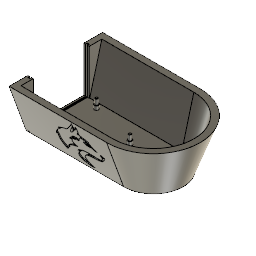
BlimpEnclosure v6 (Autodesk Fusion 360 design; units mm, degrees)
Autodesk Fusion 360 part; units mm, degrees
sketch "Sketch1" plane through (0, 0, 0) normal (0, 0, 1) x (1, 0, 0)
  line L0 (0, -53.3) -> (0, 0)
  circle A0 centre (15.3, -2.6) radius 1.4
  circle A1 centre (14, -50.8) radius 1.4
  circle A2 centre (66.1, -17.8) radius 1.4
  circle A3 centre (66.1, -45.7) radius 1.4
  line L1 (100, -58.3) -> (0, -58.3)
  line L2 (0, -58.3) -> (0, 5)
  line L3 (0, 5) -> (100, 5)
  line L4 (100, 5) -> (100, -58.3)
  line L5 (100, -58.3) -> (0, 5) construction
  line L6 (0, -58.3) -> (100, 5) construction
  arc A4 (100, -58.3) -> (100, 5) centre (100, -26.65) ccw
  line L7 (2, 3) -> (100, 3)
  arc A5 (100, -56.3) -> (100, 3) centre (100, -26.65) ccw
  line L8 (100, -56.3) -> (2, -56.3)
  line L9 (2, -56.3) -> (2, 3)
  line L10 (2, 3) -> (2, 5)
  line L11 (2, -56.3) -> (2, -58.3)
  point P0 (50, -26.65)
  dimension "d3" = 2.8
  dimension "d7" = 2.8
  dimension "d8" = 2.8
  dimension "d9" = 2.8
  dimension "d19" = 100
  dimension "d20" = 63.3
  dimension "d21" = 2
  constraint vertical L0
  constraint coincident L0.end origin
  constraint perpendicular L1 L2
  constraint parallel L1 L3
  constraint parallel L2 L4
  constraint horizontal L1
  constraint coincident L5 P0
  constraint coincident L6 P0
  constraint tangent L1 A4
  constraint coincident L3 L10.end
  constraint perpendicular L3 L10
  constraint coincident L1 L11.end
  constraint perpendicular L1 L11
  measures "d3" diameter of A0
  measures "d7" diameter of A1
  measures "d8" diameter of A2
  measures "d9" diameter of A3
  measures "d19" distance of L2.end L3.end
  measures "d20" distance of L1.end L2.end
extrude "Extrude1" add sketch "Sketch1" along normal blind 2 contours L4 L7 L8 L9 | L4 A5 makes body 1
extrude "Extrude2" add sketch "Sketch1" along normal blind 12 contours A0 | A1 | A2 | A3 bodies 1
sketch "Sketch2" plane through (0, 0, 2) normal (0, 0, 1) x (-1, 0, 0)
  circle A0 centre (-15.3, 2.6) radius 1.4
  circle A1 centre (-66.1, 17.8) radius 1.4
  circle A2 centre (-14, 50.8) radius 1.4
  circle A3 centre (-66.1, 45.7) radius 1.4
  arc A4 (-100, 56.3) -> (-100, -3) centre (-100, 26.65) ccw
  line L0 (-100, -3) -> (-2, -3)
  line L1 (-2, -3) -> (-2, 56.3)
  line L2 (-2, 56.3) -> (-100, 56.3)
  circle A5 centre (-15.3, 2.6) radius 2.25
  circle A6 centre (-66.1, 17.8) radius 2.25
  circle A7 centre (-66.1, 45.7) radius 2.25
  circle A8 centre (-14, 50.8) radius 2.25
  dimension "d26" = 4.5
  dimension "d27" = 4.5
  dimension "d28" = 4.5
  dimension "d29" = 4.5
  constraint concentric A0 A5
  constraint concentric A1 A6
  constraint concentric A3 A7
  constraint concentric A2 A8
  measures "d26" diameter of A5
  measures "d27" diameter of A6
  measures "d28" diameter of A7
  measures "d29" diameter of A8
extrude "Extrude3" add sketch "Sketch2" along normal blind 4 separate body contours A5 | A6 | A7 | A8 makes body 2 at (68.2143, -46.4695, 4.6667) makes body 3 at (11.7612, -50.576, 4.6667) makes body 4 at (63.8612, -17.576, 4.6667) makes body 5 at (13.0612, -2.376, 4.6667)
chamfer "Chamfer1" distance 0.4 angle 45 4 edges at (13.9947, -3.1063, 12) (64.7947, -18.3063, 12) (64.7947, -46.2063, 12) (12.6947, -51.3063, 12) on bodies 1
extrude "Extrude4" add sketch "Sketch1" along normal blind 50 separate body contours L1 L4 L8 L11 | L3 L4 L7 L10 | L4 A4 A5 makes body 6
draft "Draft1" angle 20 neutral plane through (0, 0, 0) pull (0, 0, -1) 3 faces at (115.1367, 1.1457, 16.6667) (34.6667, 5, 16.6667) (67.3333, -58.3, 16.6667) on bodies 6
extrude "Extrude5" add sketch "Sketch1" along normal blind 1 contours L0 L1 L2 L3 L9 L10 L11 bodies 1 6
extrude "Extrude6" add 1 faces at (2, -63.0328, 34) along direction (-1, 0, 0) blind 4 separate body on bodies 1 makes body 7
extrude "Extrude7" add 1 faces at (0, -37.2, 0.3333) along direction (-1, 0, 0) blind 2 separate body on bodies 1 makes body 8
extrude "Extrude8" cut 1 faces at (1.3333, -37.2, 1) along direction (0, 0, 1) blind 49 on bodies 1 bodies 7
draft "Draft2" angle -15 neutral plane through (0, 0, 0) pull (0, 0, -1) 3 faces at (102.9522, 2.8527, 34) (67.3333, -56.3, 18) (34.6667, 3, 18) on bodies 1
extrude "Extrude9" add 1 faces at (1.3333, -37.2, 1) along direction (0, 0, 1) blind 49 on bodies 1 bodies 1 7 8
extrude "Extrude10" add 1 faces at (-2, -63.0328, 34) along direction (-1, 0, 0) blind 2 on bodies 1 bodies 1
sketch "Sketch3" plane through (0, 0, 50) normal (0, 0, 1) x (-1, 0, 0)
  line L0 (4, 76.4985) -> (-100, 76.4985)
  arc A0 (-100, 76.4985) -> (-100, -23.1985) centre (-100, 26.65) ccw
  line L1 (-100, -23.1985) -> (4, -23.1985)
  line L2 (4, -23.1985) -> (4, -3)
  line L3 (4, -3) -> (0, -3)
  line L4 (0, -3) -> (0, 56.3)
  line L5 (0, 56.3) -> (4, 56.3)
  line L6 (4, 56.3) -> (4, 76.4985)
  line L7 (-2, 69.6975) -> (-2, -16.3975)
  line L8 (-2, -16.3975) -> (-100, -16.3975)
  arc A1 (-100, 69.6975) -> (-100, -16.3975) centre (-100, 26.65) ccw
  line L9 (-100, 69.6975) -> (-2, 69.6975)
  line L10 (0, -3) -> (-2, -3)
  line L11 (0, 56.3) -> (-2, 56.3)
  line L12 (2, -5) -> (0, -5)
  line L13 (0, -5) -> (0, 58)
  line L14 (0, 58) -> (2, 58)
  line L15 (2, 58) -> (2, -5)
  point P0 (-2, -3)
  point P1 (-2, 56.3)
  constraint coincident L3.end L4.start
  constraint coincident P0 L10.end
  constraint coincident L4.end L5.start
  constraint coincident P1 L11.end
  constraint horizontal L12
  constraint vertical L13
  constraint horizontal L14
  constraint vertical L15
sketch "Sketch4" plane through (0, 0, 50) normal (0, 0, 1) x (-1, 0, 0)
  line L0 (4, 76.4985) -> (-100, 76.4985)
  arc A0 (-100, 76.4985) -> (-100, -23.1985) centre (-100, 26.65) ccw
  line L1 (-100, -23.1985) -> (4, -23.1985)
  line L2 (4, -23.1985) -> (4, -3)
  line L3 (4, -3) -> (0, -3)
  line L4 (0, -3) -> (0, 56.3)
  line L5 (0, 56.3) -> (4, 56.3)
  line L6 (4, 56.3) -> (4, 76.4985)
  line L7 (-2, 69.6975) -> (-2, -16.3975)
  line L8 (-2, -16.3975) -> (-100, -16.3975)
  arc A1 (-100, 69.6975) -> (-100, -16.3975) centre (-100, 26.65) ccw
  line L9 (-100, 69.6975) -> (-2, 69.6975)
sketch "Sketch5" plane through (2, 0, 0) normal (1, 0, 0) x (0, 1, 0)
  line L0 (3.5359, 2) -> (16.3975, 50)
  line L1 (16.3975, 50) -> (-69.6975, 50)
  line L2 (-69.6975, 50) -> (-56.8359, 2)
  line L3 (-56.8359, 2) -> (3.5359, 2)
  line L4 (3, 50) -> (3, 2)
  line L5 (-56.3, 50) -> (-56, 2)
  line L6 (3, 50) -> (-56.3, 50)
  line L7 (3, 2) -> (-56, 2)
  line L8 (3, 50) -> (-56.3, 50)
  line L9 (-56.3, 50, -2) -> (3, 50, -2)
  line L10 (3, 50, -2) -> (3, 2, 0)
  point P0 (3, 50)
  point P1 (-56.3, 50)
  point P2 (-56.3, 50)
  point P3 (3, 50)
  constraint coincident P3 P0
  constraint coincident L3 L4.end
  constraint coincident P2 P1
  constraint coincident L3 L5.end
sketch "Sketch6" plane through (0, 0, 50) normal (0, 0, 1) x (-1, 0, 0)
  line L0 (4, 76.4985) -> (-100, 76.4985)
  arc A0 (-100, 76.4985) -> (-100, -23.1985) centre (-100, 26.65) ccw
  line L1 (-100, -23.1985) -> (4, -23.1985)
  line L2 (4, -23.1985) -> (4, -3)
  line L3 (4, -3) -> (0, -3)
  line L4 (0, -3) -> (0, 56.3)
  line L5 (0, 56.3) -> (4, 56.3)
  line L6 (4, 56.3) -> (4, 76.4985)
  line L7 (-2, 69.6975) -> (-2, -16.3975)
  line L8 (-2, -16.3975) -> (-100, -16.3975)
  arc A1 (-100, 69.6975) -> (-100, -16.3975) centre (-100, 26.65) ccw
  line L9 (-100, 69.6975) -> (-2, 69.6975)
  line L10 (-2, 56.3) -> (0, 56.3)
  line L11 (0, 56.3) -> (0, -3)
  line L12 (0, -3) -> (-2, -3)
  line L13 (-2, -3) -> (-2, 56.3)
  point P0 (-2, 56.3)
  constraint horizontal L10
  constraint vertical L11
  constraint horizontal L12
  constraint vertical L13
  constraint coincident L3.end L4.start
  constraint coincident P0 L10.start
extrude "Extrude11" cut sketch "Sketch6" against normal blind 48 contours L4 L7 L10 L11 L12 L13 bodies 1
sketch "Sketch7" plane through (0, 0, 2) normal (0, 0, 1) x (-1, 0, 0)
  circle A0 centre (-66.1, 17.8) radius 1.4
  circle A1 centre (-14, 50.8) radius 1.4
  circle A2 centre (-15.3, 2.6) radius 1.4
  circle A3 centre (-66.1, 45.7) radius 1.4
  line L0 (-2, -3) -> (4, -3)
  line L1 (4, -3) -> (4, 56.3)
  line L2 (4, 56.3) -> (-2, 56.3)
  line L3 (-2, 56.3) -> (-2, 56.8359)
  line L4 (-2, 56.8359) -> (-100, 56.8359)
  arc A4 (-100, 56.8359) -> (-100, -3.5359) centre (-100, 26.65) ccw
  line L5 (-100, -3.5359) -> (-2, -3.5359)
  line L6 (-2, -3.5359) -> (-2, -3)
  line L7 (2, -3) -> (0, -3)
  line L8 (0, -3) -> (0, 56.3)
  line L9 (0, 56.3) -> (2, 56.3)
  line L10 (2, 56.3) -> (2, -3)
  line L11 (4, -3) -> (0, -3)
  point P0 (0, 56.3)
  constraint horizontal L7
  constraint vertical L8
  constraint horizontal L9
  constraint vertical L10
  constraint coincident P0 L8.end
  constraint midpoint L7.start L11
sketch "Sketch8" plane through (0, 0, 2) normal (0, 0, 1) x (-1, 0, 0)
  circle A0 centre (-66.1, 17.8) radius 1.4
  circle A1 centre (-14, 50.8) radius 1.4
  circle A2 centre (-15.3, 2.6) radius 1.4
  circle A3 centre (-66.1, 45.7) radius 1.4
  line L0 (-2, -3) -> (4, -3)
  line L1 (4, -3) -> (4, 56.3)
  line L2 (4, 56.3) -> (-2, 56.3)
  line L3 (-2, 56.3) -> (-2, 56.8359)
  line L4 (-2, 56.8359) -> (-100, 56.8359)
  arc A4 (-100, 56.8359) -> (-100, -3.5359) centre (-100, 26.65) ccw
  line L5 (-100, -3.5359) -> (-2, -3.5359)
  line L6 (-2, -3.5359) -> (-2, -3)
  point P0 (0, -3)
  point P1 (0, 56.3)
sketch "Sketch9" plane through (0, 0, 0) normal (1, 0, 0) x (0, 1, 0)
sketch "Sketch10" plane through (0, 0, 0) normal (0, 0, 1) x (1, 0, 0)
  line L0 (-2, 5) -> (0, 5)
  line L1 (0, 5) -> (0, -58)
  line L2 (0, -58) -> (-2, -58)
  line L3 (-2, -58) -> (-2, 5)
  point P0 (-2, 5)
  point P1 (0, -58)
  constraint horizontal L0
  constraint vertical L1
  constraint horizontal L2
  constraint vertical L3
  constraint coincident P1 L1.end
  constraint coincident P0 L0.start
extrude "Extrude12" cut sketch "Sketch3" against normal blind 49 contours L3 L12 L13 L15 bodies 1
sketch "Sketch11" plane through (0, 0, 50) normal (0, 0, 1) x (-1, 0, 0)
  line L0 (2, -3) -> (2, -5)
  line L1 (2, -5) -> (0, -5)
  line L2 (0, -5) -> (0, -3)
  line L3 (0, -3) -> (-2, -3)
  line L4 (-2, -3) -> (-2, -16.3975)
  line L5 (-2, -16.3975) -> (-100, -16.3975)
  arc A0 (-100, 69.6975) -> (-100, -16.3975) centre (-100, 26.65) ccw
  line L6 (-100, 69.6975) -> (-2, 69.6975)
  line L7 (-2, 69.6975) -> (-2, 56.3)
  line L8 (-2, 56.3) -> (4, 56.3)
  line L9 (4, 56.3) -> (4, 76.4985)
  line L10 (4, 76.4985) -> (-100, 76.4985)
  arc A1 (-100, 76.4985) -> (-100, -23.1985) centre (-100, 26.65) ccw
  line L11 (-100, -23.1985) -> (4, -23.1985)
  line L12 (4, -23.1985) -> (4, -3)
  line L13 (4, -3) -> (2, -3)
extrude "Extrude13" cut sketch "Sketch7" against normal blind 1 contours L0 L2 L7 L8 L9 L10 L11 bodies 1
sketch "Sketch12" plane through (0, 0, 50) normal (0, 0, 1) x (-1, 0, 0)
  line L0 (2, -3) -> (2, -5)
  line L1 (2, -5) -> (0, -5)
  line L2 (0, -5) -> (0, -3)
  line L3 (0, -3) -> (-2, -3)
  line L4 (-2, -3) -> (-2, -16.3975)
  line L5 (-2, -16.3975) -> (-100, -16.3975)
  arc A0 (-100, 69.6975) -> (-100, -16.3975) centre (-100, 26.65) ccw
  line L6 (-100, 69.6975) -> (-2, 69.6975)
  line L7 (-2, 69.6975) -> (-2, 56.3)
  line L8 (-2, 56.3) -> (4, 56.3)
  line L9 (4, 56.3) -> (4, 76.4985)
  line L10 (4, 76.4985) -> (-100, 76.4985)
  arc A1 (-100, 76.4985) -> (-100, -23.1985) centre (-100, 26.65) ccw
  line L11 (-100, -23.1985) -> (4, -23.1985)
  line L12 (4, -23.1985) -> (4, -3)
  line L13 (4, -3) -> (2, -3)
  line L14 (0, 56.3) -> (0, 58.3)
  line L15 (-100, 58.3) -> (4, 58.3)
  line L16 (0, 58.3) -> (2, 58.3)
  line L17 (2, 56.3) -> (2, 58.3)
  line L18 (2, 56.3) -> (0, 56.3)
  line L19 (0, 56.3) -> (0, 58.3)
  line L20 (0, 58.3) -> (2, 58.3)
  line L21 (2, 58.3) -> (2, 56.3)
  point P0 (0, 56.3)
  point P1 (0, 58.3)
  point P2 (2, 56.3)
  constraint coincident P0 L14.start
  constraint coincident P1 L14.end
  constraint coincident L15 L16.end
  constraint perpendicular L7 L16
  constraint coincident P2 L17.start
  constraint horizontal L18
  constraint vertical L19
  constraint horizontal L20
  constraint vertical L21
extrude "Extrude14" cut sketch "Sketch12" against normal blind 49 contours L8 L14 L15 L16 L17 L18 L19 L20 L21 bodies 1
sketch "Sketch13" plane through (0, -51.4802, -18.7373) normal (0, -0.939693, -0.34202) x (1, 0, 0)
  line L0 (-4, 19.9398) -> (100, 19.9398)
  line L1 (100, 19.9398) -> (100, 73.1487)
  line L2 (100, 73.1487) -> (-4, 73.1487)
  line L3 (-4, 73.1487) -> (-4, 19.9398)
  spline S0 degree 3 poles (66.4906, 23.829) (62.3965, 24.2928) (59.5622, 25.3688) (57.7413, 27.1506) knots 0 0 0 0 1 1 1 1
  spline S1 degree 3 poles (57.7413, 27.1506) (55.812, 29.0384) (55.4628, 30.9667) (56.6345, 33.2633) knots 0 0 0 0 1 1 1 1
  spline S2 degree 3 poles (56.6345, 33.2633) (57.1599, 34.2932) (59.0504, 36.2138) (60.0953, 36.7791) knots 0 0 0 0 1 1 1 1
  spline S3 degree 3 poles (60.0953, 36.7791) (60.7076, 37.1104) (60.7253, 37.1501) (60.2911, 37.2178) knots 0 0 0 0 1 1 1 1
  spline S4 degree 3 poles (60.2911, 37.2178) (59.8809, 37.2819) (58.6195, 36.9207) (56.9537, 36.2622) knots 0 0 0 0 1 1 1 1
  spline S5 degree 3 poles (56.9537, 36.2622) (56.5704, 36.1107) (56.5868, 36.1693) (57.0659, 36.6642) knots 0 0 0 0 1 1 1 1
  spline S6 degree 3 poles (57.0659, 36.6642) (58.0061, 37.6351) (60.2075, 38.8181) (62.3535, 39.5055) knots 0 0 0 0 1 1 1 1
  spline S7 degree 3 poles (62.3535, 39.5055) (65.5103, 40.5167) (67.7118, 40.7272) (72.7737, 40.5015) knots 0 0 0 0 1 1 1 1
  spline S8 degree 3 poles (72.7737, 40.5015) (80.3959, 40.1618) (81.7012, 40.2086) (82.9906, 40.8681) knots 0 0 0 0 1 1 1 1
  spline S9 degree 3 poles (82.9906, 40.8681) (85.3638, 42.082) (86.2873, 44.732) (84.8911, 46.3222) knots 0 0 0 0 1 1 1 1
  spline S10 degree 3 poles (84.8911, 46.3222) (84.5209, 46.7439) (84.2179, 47.1433) (84.2179, 47.2097) knots 0 0 0 0 1 1 1 1
  spline S11 degree 3 poles (84.2179, 47.2097) (84.2179, 47.2762) (84.5068, 47.394) (84.8599, 47.4716) knots 0 0 0 0 1 1 1 1
  spline S12 degree 3 poles (84.8599, 47.4716) (85.5892, 47.6318) (87.7043, 46.8028) (88.2493, 46.1433) knots 0 0 0 0 1 1 1 1
  spline S13 degree 3 poles (88.2493, 46.1433) (88.5439, 45.7867) (88.4984, 45.5963) (87.812, 44.3116) knots 0 0 0 0 1 1 1 1
  spline S14 degree 3 poles (87.812, 44.3116) (86.7906, 42.3999) (85.3099, 40.5449) (84.2402, 39.837) knots 0 0 0 0 1 1 1 1
  spline S15 degree 3 poles (84.2402, 39.837) (82.7235, 38.8333) (81.4811, 38.6129) (73.5591, 37.9421) knots 0 0 0 0 1 1 1 1
  spline S16 degree 3 poles (73.5591, 37.9421) (68.293, 37.4963) (65.3173, 36.2119) (63.8841, 33.7662) knots 0 0 0 0 1 1 1 1
  spline S17 degree 3 poles (63.8841, 33.7662) (63.1445, 32.5043) (63.1201, 30.9673) (63.8179, 29.5993) knots 0 0 0 0 1 1 1 1
  spline S18 degree 3 poles (63.8179, 29.5993) (64.5213, 28.2203) (66.9959, 25.8437) (68.9028, 24.7157) knots 0 0 0 0 1 1 1 1
  spline S19 degree 3 poles (68.9028, 24.7157) (69.7976, 24.1864) (70.5297, 23.7144) (70.5297, 23.6668) knots 0 0 0 0 1 1 1 1
  spline S20 degree 3 poles (70.5297, 23.6668) (70.5297, 23.5312) (68.3441, 23.619) (66.4906, 23.829) knots 0 0 0 0 1 1 1 1
  spline S21 degree 3 poles (43.014, 30.5926) (39.7927, 33.9837) (38.1636, 37.76) (38.1497, 41.8685) knots 0 0 0 0 1 1 1 1
  spline S22 degree 3 poles (38.1497, 41.8685) (38.1459, 42.9793) (38.2167, 44.1153) (38.307, 44.393) knots 0 0 0 0 1 1 1 1
  spline S23 degree 3 poles (38.307, 44.393) (38.5213, 45.0521) (38.2597, 45.0309) (37.4359, 44.3224) knots 0 0 0 0 1 1 1 1
  spline S24 degree 3 poles (37.4359, 44.3224) (37.0682, 44.0063) (36.734, 43.8478) (36.6931, 43.9703) knots 0 0 0 0 1 1 1 1
  spline S25 degree 3 poles (36.6931, 43.9703) (36.5759, 44.3221) (37.7635, 47.1409) (38.5515, 48.381) knots 0 0 0 0 1 1 1 1
  spline S26 degree 3 poles (38.5515, 48.381) (39.4827, 49.8465) (41.5322, 52.0522) (42.7335, 52.8816) knots 0 0 0 0 1 1 1 1
  line L4 (42.7335, 52.8816) -> (43.6829, 53.5372)
  line L5 (43.6829, 53.5372) -> (42.6888, 53.6494)
  line L6 (42.6888, 53.6494) -> (41.6947, 53.7615)
  line L7 (41.6947, 53.7615) -> (42.7275, 54.4789)
  spline S27 degree 3 poles (42.7275, 54.4789) (45.0138, 56.0668) (50.8992, 58.5861) (52.3223, 58.5861) knots 0 0 0 0 1 1 1 1
  spline S28 degree 3 poles (52.3223, 58.5861) (52.6495, 58.5861) (53.3517, 59.3292) (54.7081, 61.1106) knots 0 0 0 0 1 1 1 1
  spline S29 degree 3 poles (54.7081, 61.1106) (55.7654, 62.499) (57.2911, 64.4428) (58.0986, 65.4302) knots 0 0 0 0 1 1 1 1
  spline S30 degree 3 poles (58.0986, 65.4302) (58.9062, 66.4175) (59.8974, 67.8731) (60.3014, 68.6648) knots 0 0 0 0 1 1 1 1
  line L8 (60.3014, 68.6648) -> (61.0359, 70.1041)
  line L9 (61.0359, 70.1041) -> (61.677, 68.7938)
  spline S31 degree 3 poles (61.677, 68.7938) (62.2375, 67.6481) (62.3194, 67.223) (62.3287, 65.4106) knots 0 0 0 0 1 1 1 1
  spline S32 degree 3 poles (62.3287, 65.4106) (62.3373, 63.7177) (62.3937, 63.3827) (62.6361, 63.5835) knots 0 0 0 0 1 1 1 1
  spline S33 degree 3 poles (62.6361, 63.5835) (63.0885, 63.9582) (63.8172, 65.4801) (64.3798, 67.2254) knots 0 0 0 0 1 1 1 1
  line L10 (64.3798, 67.2254) -> (64.8861, 68.7962)
  line L11 (64.8861, 68.7962) -> (65.4055, 67.6742)
  spline S34 degree 3 poles (65.4055, 67.6742) (65.8666, 66.678) (65.9252, 66.2133) (65.9272, 63.531) knots 0 0 0 0 1 1 1 1
  line L12 (65.9272, 63.531) -> (65.9296, 60.5098)
  line L13 (65.9296, 60.5098) -> (64.9198, 60.2992)
  line L14 (64.9198, 60.2992) -> (63.91, 60.0886)
  line L15 (63.91, 60.0886) -> (65.9296, 59.6837)
  spline S35 degree 3 poles (65.9296, 59.6837) (68.232, 59.222) (71.8445, 58.1197) (73.6014, 57.3427) knots 0 0 0 0 1 1 1 1
  spline S36 degree 3 poles (73.6014, 57.3427) (74.4034, 56.988) (74.794, 56.6831) (74.7954, 56.4106) knots 0 0 0 0 1 1 1 1
  spline S37 degree 3 poles (74.7954, 56.4106) (74.8, 55.5692) (75.9, 53.6888) (77.0638, 52.5329) knots 0 0 0 0 1 1 1 1
  spline S38 degree 3 poles (77.0638, 52.5329) (77.728, 51.8732) (79.0287, 50.8448) (79.9544, 50.2475) knots 0 0 0 0 1 1 1 1
  spline S39 degree 3 poles (79.9544, 50.2475) (80.88, 49.6502) (81.5164, 49.1615) (81.3686, 49.1614) knots 0 0 0 0 1 1 1 1
  spline S40 degree 3 poles (81.3686, 49.1614) (81.2208, 49.1614) (80.2326, 49.4752) (79.1726, 49.8588) knots 0 0 0 0 1 1 1 1
  spline S41 degree 3 poles (79.1726, 49.8588) (76.7782, 50.7252) (74.8957, 52.0858) (73.6526, 53.8486) knots 0 0 0 0 1 1 1 1
  spline S42 degree 3 poles (73.6526, 53.8486) (72.6279, 55.3016) (71.8019, 55.7921) (69.2683, 56.452) knots 0 0 0 0 1 1 1 1
  spline S43 degree 3 poles (69.2683, 56.452) (67.4834, 56.9169) (66.4433, 56.8826) (65.7484, 56.3361) knots 0 0 0 0 1 1 1 1
  spline S44 degree 3 poles (65.7484, 56.3361) (64.9965, 55.7446) (63.9011, 53.8176) (63.5317, 52.4367) knots 0 0 0 0 1 1 1 1
  line L16 (63.5317, 52.4367) -> (63.24, 51.3459)
  line L17 (63.24, 51.3459) -> (61.2363, 51.4881)
  spline S45 degree 3 poles (61.2363, 51.4881) (60.0693, 51.571) (58.382, 51.5177) (57.1956, 51.3605) knots 0 0 0 0 1 1 1 1
  line L18 (57.1956, 51.3605) -> (55.1585, 51.0906)
  line L19 (55.1585, 51.0906) -> (56.2805, 50.9028)
  spline S46 degree 3 poles (56.2805, 50.9028) (57.9134, 50.6294) (59.0855, 50.2906) (59.0855, 50.0919) knots 0 0 0 0 1 1 1 1
  spline S47 degree 3 poles (59.0855, 50.0919) (59.0855, 49.9965) (58.6058, 49.8964) (58.0196, 49.8695) knots 0 0 0 0 1 1 1 1
  spline S48 degree 3 poles (58.0196, 49.8695) (55.9941, 49.7764) (53.6328, 48.8972) (52.2414, 47.718) knots 0 0 0 0 1 1 1 1
  line L20 (52.2414, 47.718) -> (51.5682, 47.1475)
  line L21 (51.5682, 47.1475) -> (52.5501, 47.4813)
  spline S49 degree 3 poles (52.5501, 47.4813) (53.934, 47.9517) (54.692, 47.9286) (54.485, 47.4223) knots 0 0 0 0 1 1 1 1
  spline S50 degree 3 poles (54.485, 47.4223) (54.3967, 47.2064) (54.2255, 46.6864) (54.1046, 46.2669) knots 0 0 0 0 1 1 1 1
  spline S51 degree 3 poles (54.1046, 46.2669) (53.6035, 44.5285) (54.9864, 42.386) (57.1364, 41.5699) knots 0 0 0 0 1 1 1 1
  line L22 (57.1364, 41.5699) -> (58.1844, 41.1721)
  line L23 (58.1844, 41.1721) -> (56.0154, 40.5625)
  spline S52 degree 3 poles (56.0154, 40.5625) (53.3032, 39.8001) (50.1984, 38.3321) (48.3738, 36.9494) knots 0 0 0 0 1 1 1 1
  spline S53 degree 3 poles (48.3738, 36.9494) (47.1179, 35.9975) (45.762, 34.5849) (45.9367, 34.4102) knots 0 0 0 0 1 1 1 1
  spline S54 degree 3 poles (45.9367, 34.4102) (45.9735, 34.3734) (46.4478, 34.5448) (46.9907, 34.7911) knots 0 0 0 0 1 1 1 1
  spline S55 degree 3 poles (46.9907, 34.7911) (48.6211, 35.5308) (48.6243, 35.3215) (47.006, 33.7949) knots 0 0 0 0 1 1 1 1
  spline S56 degree 3 poles (47.006, 33.7949) (46.0793, 32.9207) (45.1776, 31.8023) (44.7446, 30.9899) knots 0 0 0 0 1 1 1 1
  spline S57 degree 3 poles (44.7446, 30.9899) (44.3486, 30.2469) (44.0009, 29.6389) (43.9722, 29.6389) knots 0 0 0 0 1 1 1 1
  spline S58 degree 3 poles (43.9722, 29.6389) (43.9434, 29.6389) (43.5122, 30.0681) (43.014, 30.5926) knots 0 0 0 0 1 1 1 1
  line L24 (43.014, 30.5926) -> (43.014, 30.5926)
  spline S59 degree 3 poles (58.7431, 59.1951) (59.7873, 59.803) (59.8912, 59.947) (60.3559, 61.4308) knots 0 0 0 0 1 1 1 1
  spline S60 degree 3 poles (60.3559, 61.4308) (60.6291, 62.303) (60.9142, 63.9132) (60.9896, 65.0088) knots 0 0 0 0 1 1 1 1
  spline S61 degree 3 poles (60.9896, 65.0088) (61.1236, 66.9576) (61.1184, 66.9863) (60.7509, 66.3278) knots 0 0 0 0 1 1 1 1
  spline S62 degree 3 poles (60.7509, 66.3278) (60.5443, 65.9575) (59.717, 64.5555) (58.9125, 63.2122) knots 0 0 0 0 1 1 1 1
  spline S63 degree 3 poles (58.9125, 63.2122) (57.7333, 61.2432) (56.3927, 58.2111) (56.3927, 57.5128) knots 0 0 0 0 1 1 1 1
  spline S64 degree 3 poles (56.3927, 57.5128) (56.3927, 57.4398) (56.6704, 57.6423) (57.0098, 57.9627) knots 0 0 0 0 1 1 1 1
  spline S65 degree 3 poles (57.0098, 57.9627) (57.3492, 58.2832) (58.1292, 58.8377) (58.7431, 59.1951) knots 0 0 0 0 1 1 1 1
  spline S66 degree 3 poles (71.3151, 51.0838) (70.9449, 51.2757) (70.3342, 51.7295) (69.9581, 52.0922) knots 0 0 0 0 1 1 1 1
  spline S67 degree 3 poles (69.9581, 52.0922) (69.5819, 52.455) (69.1275, 52.7533) (68.9483, 52.7552) knots 0 0 0 0 1 1 1 1
  spline S68 degree 3 poles (68.9483, 52.7552) (68.769, 52.757) (68.4709, 52.8641) (68.2858, 52.9931) knots 0 0 0 0 1 1 1 1
  spline S69 degree 3 poles (68.2858, 52.9931) (68.0447, 53.161) (68.5544, 53.2038) (70.0809, 53.1438) knots 0 0 0 0 1 1 1 1
  spline S70 degree 3 poles (70.0809, 53.1438) (72.1426, 53.0628) (72.2385, 53.0354) (72.9981, 52.3105) knots 0 0 0 0 1 1 1 1
  spline S71 degree 3 poles (72.9981, 52.3105) (73.4301, 51.8983) (74.0864, 51.3749) (74.4567, 51.1474) knots 0 0 0 0 1 1 1 1
  line L25 (74.4567, 51.1474) -> (75.1299, 50.7339)
  line L26 (75.1299, 50.7339) -> (73.5591, 50.7343)
  spline S72 degree 3 poles (73.5591, 50.7343) (72.5776, 50.7347) (71.7358, 50.8657) (71.3151, 51.0837) knots 0 0 0 0 1 1 1 1
  line L27 (71.3151, 51.0837) -> (71.3151, 51.0838)
extrude "Extrude15" cut sketch "Sketch13" against normal blind 1 contours S0 S1 S2 S3 S4 S5 S6 S7 S8 S9 S10 S11 S12 S13 S14 S15 S16 S17 S18 S19 S20 | S21 S22 S23 S24 S25 S26 L4 L5 L6 L7 S27 S28 S29 S30 L8 L9 S31 S32 S33 L10 L11 S34 L12 L13 L14 L15 S35 S36 S37 S38 S39 S40 S41 S42 S43 S44 L16 L17 S45 L18 L19 S46 S47 S48 L20 L21 S49 S50 S51 L22 L23 S52 S53 S54 S55 S56 S57 S58 | S66 S67 S68 S69 S70 S71 L25 L26 S72 bodies 1
sketch "Sketch14" plane through (0, 4.4151, -1.607) normal (0, 0.939693, -0.34202) x (-1, 0, 0)
  line L0 (-100, 1.7101) -> (4, 1.7101)
  line L1 (4, 1.7101) -> (4, 54.919)
  line L2 (4, 54.919) -> (-100, 54.919)
  line L3 (-100, 54.919) -> (-100, 1.7101)
  line L4 (-49.6043, 46.2383) -> (-49.6043, 37.0097)
  line L5 (-49.6043, 37.0097) -> (-45.5023, 37.0097)
  spline S0 degree 3 poles (-45.5023, 37.0097) (-46.0413, 35.0048) (-47.4095, 29.9155) (-48.6833, 25.1727) knots 0 0 0 0 1 1 1 1
  spline S1 degree 2 poles (-48.6833, 25.1727) (-50.3168, 31.7516) (-53.9154, 46.2386) knots 0 0 0 1 1 1
  line L6 (-53.9154, 46.2386) -> (-62.6157, 46.2382)
  spline S2 degree 2 poles (-62.6157, 46.2382) (-66.5081, 31.7498) (-68.2727, 25.1815) knots 0 0 0 1 1 1
  spline S3 degree 3 poles (-68.2727, 25.1815) (-69.4502, 29.9406) (-70.7101, 35.0339) (-71.1995, 37.0097) knots 0 0 0 0 1 1 1 1
  line L7 (-71.1995, 37.0097) -> (-66.8749, 37.0097)
  line L8 (-66.8749, 37.0097) -> (-66.8749, 46.2382)
  line L9 (-66.8749, 46.2382) -> (-88.5665, 46.2382)
  line L10 (-88.5665, 46.2382) -> (-88.5665, 37.0097)
  line L11 (-88.5665, 37.0097) -> (-84.0715, 37.0097)
  spline S4 degree 2 poles (-84.0715, 37.0097) (-83.5811, 35.0469) (-76.7572, 7.7505) knots 0 0 0 1 1 1
  line L12 (-76.7572, 7.7505) -> (-64.4475, 7.7501)
  spline S5 degree 2 poles (-64.4475, 7.7501) (-62.1259, 16.5756) (-60.7137, 21.9426) knots 0 0 0 1 1 1
  spline S6 degree 2 poles (-60.7137, 21.9426) (-59.371, 16.5731) (-57.1637, 7.7505) knots 0 0 0 1 1 1
  line L13 (-57.1637, 7.7505) -> (-44.8555, 7.7501)
  spline S7 degree 2 poles (-44.8555, 7.7501) (-37.6665, 35.0754) (-37.1579, 37.0097) knots 0 0 0 1 1 1
  line L14 (-37.1579, 37.0097) -> (-32.6847, 37.0097)
  line L15 (-32.6847, 37.0097) -> (-32.6847, 46.2382)
  line L16 (-32.6847, 46.2382) -> (-49.6035, 46.2382)
  line L17 (-49.6035, 46.2382) -> (-49.6043, 46.2383)
  line L18 (-48.2152, 44.8451) -> (-48.2152, 38.4065)
  line L19 (-48.2152, 38.4065) -> (-43.6902, 38.4065)
  line L20 (-43.6902, 38.4065) -> (-48.742, 19.6026)
  spline S8 degree 2 poles (-48.742, 19.6026) (-54.925, 44.4946) (-55.0128, 44.8451) knots 0 0 0 1 1 1
  line L21 (-55.0128, 44.8451) -> (-61.5525, 44.8451)
  spline S9 degree 2 poles (-61.5525, 44.8451) (-61.6446, 44.5029) (-68.3348, 19.6012) knots 0 0 0 1 1 1
  line L22 (-68.3348, 19.6012) -> (-72.988, 38.4065)
  line L23 (-72.988, 38.4065) -> (-68.2759, 38.4065)
  line L24 (-68.2759, 38.4065) -> (-68.2759, 44.8451)
  line L25 (-68.2759, 44.8451) -> (-87.1779, 44.8451)
  line L26 (-87.1779, 44.8451) -> (-87.1779, 38.4065)
  line L27 (-87.1779, 38.4065) -> (-82.9892, 38.4065)
  spline S10 degree 2 poles (-82.9892, 38.4065) (-75.762, 9.4969) (-75.675, 9.1458) knots 0 0 0 1 1 1
  line L28 (-75.675, 9.1458) -> (-65.5285, 9.1458)
  spline S11 degree 2 poles (-65.5285, 9.1458) (-65.4391, 9.4884) (-60.6857, 27.5573) knots 0 0 0 1 1 1
  spline S12 degree 2 poles (-60.6857, 27.5573) (-56.1688, 9.4943) (-56.0821, 9.1458) knots 0 0 0 1 1 1
  line L29 (-56.0821, 9.1458) -> (-45.9364, 9.1458)
  spline S13 degree 2 poles (-45.9364, 9.1458) (-45.8457, 9.4917) (-38.2399, 38.4065) knots 0 0 0 1 1 1
  line L30 (-38.2399, 38.4065) -> (-34.0861, 38.4065)
  line L31 (-34.0861, 38.4065) -> (-34.0861, 44.8451)
  line L32 (-34.0861, 44.8451) -> (-48.2152, 44.8451)
extrude "Extrude16" cut sketch "Sketch14" against normal blind 1 contours L4 L5 S0 S1 L6 S2 S3 L7 L8 L9 L10 L11 S4 L12 S5 S6 L13 S7 L14 L15 L16 | L18 L19 L20 S8 L21 S9 L22 L23 L24 L25 L26 L27 S10 L28 S11 S12 L29 S13 L30 L31 L32 bodies 1
combine "Combine1" operation add target body 1 tool bodies 2 3 4 5
copy_body "Body->Comp1" bodies 1 removing the originals makes body 9 in component "Component"
component "Component" placed x (1, 0, 0) y (0, 1, 0) z (0, 0, 1) at (0, 0, 0)
